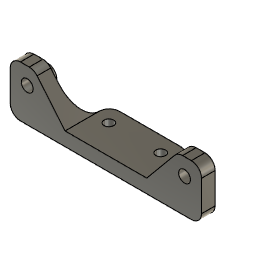
V3D ADXL mount v5 (Autodesk Fusion 360 design; units mm, degrees)
Autodesk Fusion 360 part; units mm, degrees
sketch "Sketch1" plane through (0, 0, 0) normal (0, 1, 0) x (1, 0, 0)
  line L0 (0, 0) -> (-28.109, 0)
  line L1 (-28.109, 0) -> (-28.109, -15)
  line L2 (-28.109, -15) -> (-21.109, -15)
  line L3 (-21.109, -15) -> (-12, -4)
  line L4 (-12, -4) -> (0, -4)
  line L5 (0, -4) -> (0, 0)
  circle A0 centre (-23.109, -10) radius 1.75
  line L6 (0, -1.75) -> (0, -22.5)
  line L7 (0, 0) -> (28.109, 0)
  line L8 (28.109, 0) -> (28.109, -15)
  line L9 (28.109, -15) -> (21.109, -15)
  line L10 (12, -4) -> (0, -4)
  line L11 (0, -4) -> (0, 0)
  line L12 (21.109, -15) -> (12, -4)
  circle A1 centre (23.109, -10) radius 1.75
  dimension "d1" = 23.109
  dimension "d2" = 3.5
  dimension "d3" = 10
  dimension "d4" = 5
  dimension "d5" = 5
  dimension "d6" = 7
  dimension "d8" = 12
  dimension "d9" = 4
  constraint coincident L0.start L5.end
  constraint horizontal L0
  constraint perpendicular L0 L1
  constraint perpendicular L1 L2
  constraint perpendicular L1 L4
  constraint perpendicular L4 L5
  constraint symmetric L0.start L6 L5.end
  constraint symmetric L0.end L6 L7.end
  constraint symmetric L1.end L6 L8.end
  constraint symmetric L2.end L6 L9.end
  constraint symmetric L3.end L6 L10.start
  constraint symmetric L4.end L6 L5.start
  constraint symmetric A0 L6 A1
  measures "d1" distance of L5 A0.centre
  measures "d2" diameter of A0
  measures "d3" distance of L0 A0.centre
  measures "d4" distance of L1 A0.centre
  measures "d5" distance of L2 A0.centre
  measures "d6" distance of L1.end L2.end
  measures "d8" distance of L3.end L4.end
  measures "d9" distance of L0 L4
extrude "Extrude1" add sketch "Sketch1" along normal blind 4
sketch "Sketch2" plane through (0, 4, 0) normal (0, 1, 0) x (-1, 0, 0)
  circle A0 centre (23.109, 10) radius 1.75
  circle A1 centre (-23.109, 10) radius 1.75
  line L0 (-28.109, 0) -> (28.109, 0)
  line L1 (28.109, 0) -> (28.109, 15)
  line L2 (28.109, 15) -> (21.109, 15)
  line L3 (21.109, 15) -> (12, 4)
  line L4 (12, 4) -> (-12, 4)
  line L5 (-12, 4) -> (-21.109, 15)
  line L6 (-21.109, 15) -> (-28.109, 15)
  line L7 (-28.109, 15) -> (-28.109, 0)
  line L8 (-12, 4) -> (12, 4)
  line L9 (12, 4) -> (12, 0)
  line L10 (12, 0) -> (-12, 0)
  line L11 (-12, 0) -> (-12, 4)
  constraint horizontal L8
  constraint vertical L9
  constraint horizontal L10
  constraint vertical L11
  constraint coincident L0 L9.end
  constraint coincident L4.end L5.start
  constraint coincident L3.end L4.start
extrude "Extrude2" add sketch "Sketch2" along normal blind 9 contours L0 L4 L8 L9 L10 L11
sketch "Sketch3" plane through (0, 4, 0) normal (0, 1, 0) x (-1, 0, 0)
  line L0 (12, 4) -> (12, 0)
  line L1 (12, 0) -> (28.109, 0)
  line L2 (28.109, 0) -> (28.109, 15)
  line L3 (28.109, 15) -> (21.109, 15)
  line L4 (21.109, 15) -> (12, 4)
  circle A0 centre (23.109, 10) radius 1.75
  circle A1 centre (23.109, 10) radius 3
  line L5 (-12, 0) -> (-12, 4)
  line L6 (-12, 4) -> (-21.109, 15)
  line L7 (-21.109, 15) -> (-28.109, 15)
  line L8 (-28.109, 15) -> (-28.109, 0)
  line L9 (-28.109, 0) -> (-12, 0)
  circle A2 centre (-23.109, 10) radius 1.75
  circle A3 centre (-23.109, 10) radius 3
  dimension "d14" = 6
  constraint concentric A0 A1
  constraint concentric A2 A3
  constraint equal A1 A3
  measures "d14" diameter of A3
extrude "Extrude3" add sketch "Sketch3" along normal blind 2 contours A1 | A3
chamfer "Chamfer1" distance 0.3 distance2 2 2 edges at (25.906, 6, 8.9152) (-20.312, 6, 8.9152) measured on face at (20.5434, 6, 9.764) measured on face at (-25.6746, 6, 9.764)
sketch "Sketch4" plane through (0, 0, 4) normal (0, 0, 1) x (-1, 0, 0)
  line L0 (12, 0) -> (-12, 0)
  line L1 (-12, 0) -> (-12, -4)
  line L2 (-12, -4) -> (-12, -13)
  line L3 (-12, -13) -> (12, -13)
  line L4 (12, -13) -> (12, -4)
  line L5 (12, -4) -> (12, 0)
  line L6 (0, 0) -> (0, -19.3356) construction
  circle A0 centre (7.62, -8.5) radius 1.425
  circle A1 centre (-7.62, -8.5) radius 1.425
  dimension "d19" = 7.62
  dimension "d20" = 2.85
  dimension "d21" = 8.5
  constraint coincident L6.start origin
  constraint perpendicular L3 L6
  constraint symmetric L6 A0 A1
  measures "d19" distance of L6 A0.centre
  measures "d20" diameter of A0
  measures "d21" distance of L0 A0.centre
extrude "Extrude4" cut sketch "Sketch4" against normal blind 10 contours A0 | A1
fillet "Fillet1" radius 3 8 edges at (28.109, 2, 0) (28.109, 2, 15) (21.109, 2, 15) (-21.109, 2, 15) (-28.109, 2, 15) (-28.109, 2, 0) (12, 13, 2) (-12, 13, 2)
fillet "Fillet2" radius 6 2 edges at (12, 4, 2) (-12, 4, 2)
equation "d1 = ( 46.218 / 2 ) * 1 mm"
